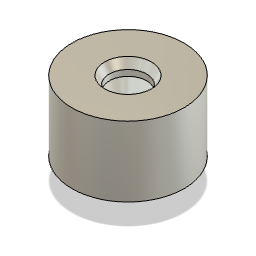
Blender_Feet_Extenders (Autodesk Fusion 360 design; units mm, degrees)
Autodesk Fusion 360 part; units mm, degrees
sketch "Sketch2" plane through (0, 0, 0) normal (0, 0, 1) x (1, 0, 0)
  line L0 (12, 15) -> (12, 0)
  line L1 (12, 0) -> (6.6, 0)
  line L2 (0, 0) -> (0, 15) construction
  line L3 (0, 15) -> (4, 15) construction
  line L4 (4, 15) -> (12, 15)
  line L5 (0, 0) -> (0, -4.5) construction
  line L6 (3, -4.5) -> (6.6, -4.5)
  line L7 (6.6, -4.5) -> (6.6, 0)
  line L8 (6.6, 0) -> (0, 0) construction
  line L9 (4, 15) -> (4, 12)
  line L10 (4, 12) -> (6.1, 12)
  line L11 (6.1, 12) -> (3, 3.4828)
  line L12 (3, 3.4828) -> (3, -4.5)
  line L13 (0, -4.5) -> (3, -4.5) construction
  dimension "d15" = 12
  dimension "d17" = 15
  dimension "d18" = 6.6
  dimension "d19" = 4
  dimension "d20" = 3
  dimension "d21" = 6.1
  dimension "d22" = 70
  dimension "d23" = 3
  dimension "d24" = 4.5
  constraint vertical L0
  constraint horizontal L1
  constraint vertical L2
  constraint coincident L2.start L5.start
  constraint perpendicular L2 L3
  constraint perpendicular L0 L4
  constraint perpendicular L1 L5
  constraint perpendicular L2 L6
  constraint perpendicular L1 L7
  constraint horizontal L8
  constraint perpendicular L3 L9
  constraint perpendicular L9 L10
  constraint perpendicular L6 L12
  constraint perpendicular L2 L13
  measures "d15" distance of L0 L2
  measures "d17" distance of L1 L4
  measures "d18" distance of L5 L7
  measures "d19" distance of L2 L3.end
  measures "d20" distance of L4 L10
  measures "d21" distance of L2 L10.end
  measures "d22" angle of L10 L11
  measures "d23" distance of L2 L12
  measures "d24" distance of L1 L6
revolve "Revolve1" add sketch "Sketch2" angle 360 about axis through (0, 0, 0) along (0, 1, 0)
chamfer "Chamfer1" distance 1 angle 60 2 edges at (-3.7293, 15, -1.4465) (-6.1534, -4.5, -2.3867) measured on face at (9.2887, 15, 0.5962) measured on face at (5.3754, -4.5, 0.3279)
